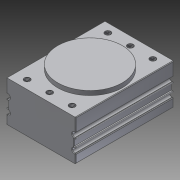
# Autodesk Inventor part: Rotary Pneumatic Cylinder Body
Saved by Autodesk Inventor 2014 SP1 (Build 180222100, 222)
## iProperties
Created: 2013-12-16
Part Number: Rotary Pneumatic Cylinder Body
Material: Generic
Document SubType Name: Modeling
Designer: Moses
Density: 1 g/cm^3
Appearance: Aluminum - Flat
Mass: 365.775 g
Surface Area: 412.742 cm^2
Volume: 365.775 cm^3
Author: Moses
Autodesk Inventor part; units mm, degrees
ref_plane "YZ Plane" through (0, 0, 0) normal (1, 0, 0) x (0, 1, 0)
ref_plane "XZ Plane" through (0, 0, 0) normal (0, 1, 0) x (-1, 0, 0)
ref_plane "XY Plane" through (0, 0, 0) normal (0, 0, 1) x (1, 0, 0)
sketch "Sketch1" plane through (0, 0, 0) normal (0, 0, 1) x (1, 0, 0)
  line L0 (0, 0) -> (0, 9.525)
  line L1 (0, 9.525) -> (1.27, 9.525)
  line L2 (1.27, 14.605) -> (0, 14.605)
  line L3 (0, 24.4475) -> (1.27, 24.4475)
  line L4 (1.27, 29.5275) -> (0, 29.5275)
  line L5 (0, 29.5275) -> (0, 44.45)
  line L6 (0, 44.45) -> (38.1, 44.45)
  line L7 (38.1, 44.45) -> (38.1, 0)
  line L8 (38.1, 0) -> (0, 0)
  arc A0 (1.27, 24.4475) -> (1.27, 29.5275) centre (1.27, 26.9875) ccw
  arc A1 (1.27, 9.525) -> (1.27, 14.605) centre (1.27, 12.065) ccw
  line L9 (0, 24.4475) -> (0, 23.1775)
  line L10 (0, 23.1775) -> (1.905, 23.1775)
  line L11 (1.905, 23.1775) -> (1.905, 15.875)
  line L12 (1.905, 15.875) -> (0, 15.875)
  line L13 (0, 15.875) -> (0, 14.605)
  dimension "d0" = 2.54
  dimension "d1" = 44.45
  dimension "d4" = 1.27
  dimension "d5" = 38.1
  dimension "d8" = 1.905
  dimension "d9" = 1.27
  dimension "d11" = 17.4625
  dimension "d12" = 12.065
  constraints: 28 end point, 7 horizontal, 6 vertical, 5 equal length, 4 point on circle, 4 tangent, 2 centre point, 1 equal radius, 1 perpendicular
  measures "d0" radius of A1
  measures "d1" distance between parallel lines of L8 L6
  measures "d4" distance of L0.end L1.end
  measures "d5" distance of L7.end L0.start
  measures "d8" distance of L11.end L12.end
  measures "d9" distance of L3.start L9.end
  measures "d11" distance from line of L6 A0.centre
  measures "d12" distance from line of L8 A1.centre
extrude "Extrusion1" add sketch "Sketch1" along normal blind 107.95
fillet "Fillet1" radius 0.635 34 edges at (0, 15.875, 53.975) (0, 14.605, 53.975) (0, 23.1775, 53.975) (0, 24.4475, 53.975) (0, 29.5275, 53.975) (0, 9.525, 53.975) (0, 0, 53.975) (0, 44.45, 53.975) (0, 36.9888, 107.95) (0.635, 24.4475, 107.95) (0.635, 29.5275, 107.95) (3.81, 26.9875, 107.95) (0, 23.8125, 107.95) (0.9525, 23.1775, 107.95) (1.905, 19.5263, 107.95) (0.9525, 15.875, 107.95) (0, 15.24, 107.95) (0.635, 9.525, 107.95) (0.635, 14.605, 107.95) (3.81, 12.065, 107.95) (0, 4.7625, 107.95) (0, 36.9888, 0) (3.81, 26.9875, 0) (0.635, 24.4475, 0) (0.635, 29.5275, 0) (0, 23.8125, 0) (0.9525, 23.1775, 0) (1.905, 19.5263, 0) (0.9525, 15.875, 0) (0, 15.24, 0) (3.81, 12.065, 0) (0.635, 9.525, 0) (0.635, 14.605, 0) (0, 4.7625, 0)
mirror "Mirror1" about plane through (38.1, 0, 0) normal (1, 0, 0)
sketch "Sketch2" plane through (0.635, 44.45, 107.95) normal (0, 1, 0) x (1, 0, 0)
  line L0 (0, 0) -> (0, 107.95) projected
  line L1 (74.93, 0) -> (74.93, 107.95) projected
  line L2 (0, 107.95) -> (74.93, 107.95) projected
  line L3 (0, 53.975) -> (74.93, 53.975) construction
  line L4 (0, 98.425) -> (74.93, 98.425) construction
  circle A0 centre (37.465, 53.975) radius 35.56
  circle A1 centre (12.7, 98.425) radius 3.175
  circle A2 centre (37.465, 98.425) radius 3.175
  circle A3 centre (62.23, 98.425) radius 3.175
  circle A4 centre (12.7, 9.525) radius 3.175
  circle A5 centre (37.465, 9.525) radius 3.175
  circle A6 centre (62.23, 9.525) radius 3.175
  point P0 (-0.635, 107.95)
  dimension "d13" = 71.12
  dimension "d14" = 9.525
  dimension "d16" = 6.35
  dimension "d19" = 24.765
  dimension "d22" = 88.9
  dimension "d25" = 107.95
  dimension "d27" = 12.7
  dimension "d28" = 74.93
  constraints: 7 centre point, 4 end point, 3 midpoint, 3 point on line, 2 horizontal, 1 vertical, 10 other
  measures "d13" diameter of A0
  measures "d14" distance between parallel lines of L2 L4
  measures "d16" diameter of A1
  measures "d19" distance of A1.centre A2.centre
  measures "d22" distance of A1.centre A4.centre
  measures "d25" distance of L0.start L0.end
  measures "d27" distance of L4.start A1.centre
  measures "d28" distance of L0.end L1.end
extrude "Extrusion2" cut sketch "Sketch2" against normal through all contours A1 | A2 | A3 | A4 | A5 | A6
extrude "Extrusion3" add sketch "Sketch2" along normal blind 4.7625 contours A0
thread "Thread1" size "1/4-20 UNC" class "2B" standard "ANSI Unified Screw Threads" full length
thread "Thread2" size "1/4-20 UNC" class "2B" standard "ANSI Unified Screw Threads" full length
thread "Thread3" size "1/4-20 UNC" class "2B" standard "ANSI Unified Screw Threads" full length
thread "Thread4" size "1/4-20 UNC" class "2B" standard "ANSI Unified Screw Threads" full length
thread "Thread5" size "1/4-20 UNC" class "2B" standard "ANSI Unified Screw Threads" full length
thread "Thread6" size "1/4-20 UNC" class "2B" standard "ANSI Unified Screw Threads" full length
equation "\"d19\" = -d27 + 0.5 * d28"
equation "\"d22\" = d25 - 2 * d14"
body "Solid1"
